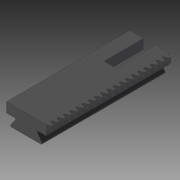
# Autodesk Inventor part: 3102_Dovetail Slider_V2
Saved by Autodesk Inventor 2021 (Build 250183000, 183)
## iProperties
Created: 2019-10-22
Part Number: 3102_Dovetail Slider_V2
Material: Acetal Resin, White
Document SubType Name: Modeling
Designer: RFLab
Density: 1.425 g/cm^3
Appearance: Smooth - White
Author: RFLab
Autodesk Inventor part; units mm, degrees
ref_plane "YZ Plane" through (0, 0, 0) normal (1, 0, 0) x (0, 1, 0)
ref_plane "XZ Plane" through (0, 0, 0) normal (0, 1, 0) x (-1, 0, 0)
ref_plane "XY Plane" through (0, 0, 0) normal (0, 0, 1) x (1, 0, 0)
sketch "Sketch1" plane through (0, 0, 0) normal (0, 0, 1) x (1, 0, 0)
  line L0 (-20, -10) -> (20, -10)
  line L1 (20, -10) -> (20, 10)
  line L2 (20, 10) -> (-20, 10)
  line L3 (-20, 10) -> (-20, -10)
  point P0 (0, 0)
  dimension "d0" = 40
  dimension "d1" = 20
  dimension "d2" = 10
  dimension "d3" = 20
  constraints: 8 end point, 2 parallel, 1 horizontal, 1 perpendicular
  measures "d0" distance of L1.end L2.end
  measures "d1" distance of L0.end L1.end
  measures "d2" distance from line of point (0, 0) L0
  measures "d3" distance from line of point (0, 0) L1
extrude "Extrusion1" add sketch "Sketch1" along normal blind 125
sketch "Sketch2" plane through (-20, 10, 0) normal (0, 1, 0) x (1, 0, 0)
  line L0 (40, 0) -> (0, 0) projected
  line L1 (13.9, 0) -> (26.1, 0)
  line L2 (26.1, 0) -> (26.1, -40.2)
  line L3 (26.1, -40.2) -> (13.9, -40.2)
  line L4 (13.9, -40.2) -> (13.9, 0)
  point P0 (20, 0)
  point P1 (26.1, 0)
  dimension "d6" = 40.2
  dimension "d7" = 12.2
  dimension "d8" = 13.9
  constraints: 8 end point, 2 parallel, 1 horizontal, 1 perpendicular, 1 point on line
  measures "d6" distance of L3.end L1.start
  measures "d7" distance of L2.end L3.end
  measures "d8" distance of L0.end L1.start
extrude "Extrusion2" cut sketch "Sketch2" against normal blind 10
sketch "Sketch4" plane through (-20, 0, 0) normal (0, 1, 0) x (1, 0, 0)
  circle A0 centre (20, -10.1) radius 1.25
  line L0 (13.9, 0) -> (26.1, 0) projected
  line L1 (13.9, -40.2) -> (13.9, 0) projected
  circle A1 centre (20, -30.1) radius 1.25
  point P0 (20, 0)
  dimension "d14" = 2.5
  dimension "d15" = 10.1
  dimension "d16" = 6.1
  dimension "d35" = 20
  dimension "d36" = 6.1
  constraints: 2 centre point, 1 equal radius
  measures "d14" diameter of A0
  measures "d15" distance from line of L0 A0.centre
  measures "d16" distance from line of L1 A0.centre
  measures "d35" distance of A1.centre A0.centre
  measures "d36" distance from line of L1 A1.centre
extrude "Extrusion4" cut sketch "Sketch4" against normal through all
sketch "Sketch5" plane through (0, 0, 125) normal (0, 0, 1) x (1, 0, 0)
  line L0 (-20, 10) -> (-20, -10) projected
  line L1 (20, -10) -> (20, 10) projected
  line L2 (-20, 0) -> (-10, 0)
  line L3 (-10, 0) -> (-20, -10)
  line L4 (-20, 0) -> (-20, -10)
  line L5 (20, 0) -> (20, -10)
  line L6 (20, 0) -> (10, 0)
  line L7 (10, 0) -> (20, -10)
  line L8 (-20, -10) -> (-17, -10)
  line L9 (-20, -10) -> (20, -10) projected
  line L10 (-10, 0) -> (-17, -10)
  line L11 (10, 0) -> (17, -10)
  line L12 (17, -10) -> (20, -10)
  point P0 (0, 0)
  point P1 (20, 5.7)
  dimension "d19" = 10
  dimension "d21" = 10
  dimension "d24" = 3
  dimension "d25" = 3
  constraints: 20 end point, 3 collinear, 2 horizontal, 2 midpoint, 2 point on line
  measures "d19" distance of L2.start L2.end
  measures "d21" distance of L5.start L6.end
  measures "d24" distance of L0.end L8.end
  measures "d25" distance of L11.end L1.start
extrude "Extrusion5" cut sketch "Sketch5" against normal through all
fillet "Fillet1" radius 1 4 edges at (17, -10, 62.5) (10, 0, 62.5) (-17, -10, 62.5) (-10, 0, 62.5)
sketch "Sketch8" plane through (-20, 10, 125) normal (0, 1, 0) x (1, 0, 0)
  line L0 (40, 125) -> (40, 0) projected
  line L1 (40, 0) -> (0, 0) projected
  line L2 (40, 0) -> (44.3156, 1.5708)
  line L3 (44.3156, 1.5708) -> (44.3156, 3.1415)
  line L4 (44.3156, 3.1415) -> (40, 4.7123)
  line L5 (40, 0) -> (40, 6.283)
  point P0 (20, 125)
  dimension "d51" = 110
  dimension "d52" = 70
  dimension "d53" = 1.5708
  dimension "d54" = 6.283
  dimension "d55" = 1.5708
  constraints: 8 end point, 2 point on line, 1 vertical
  measures "d51" angle of L0 L4
  measures "d52" angle of L0 L2
  measures "d53" distance of L2.end L3.end
  measures "d54" distance from line of L1 L5.end
  measures "d55" distance of L5.end L4.end
extrude "Extrusion8" add sketch "Sketch8" against normal blind 5
pattern_linear "Rectangular Pattern2" count 20 spacing 6.283 along (0, 0, -1) of "Extrusion8"
equation "\"d2\" = 0.5 * d1"
equation "\"d3\" = 0.5 * d0"
equation "\"d55\" = d53"
body "Solid1"
